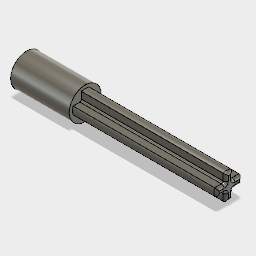
coupler2.0 v6 (Autodesk Fusion 360 design; units mm, degrees)
Autodesk Fusion 360 part; units mm, degrees
sketch "Sketch1" plane through (0, 0, 0) normal (1, 0, 0) x (0, 0, -1)
  circle A0 centre (0, 0) radius 2.3995
  dimension "d1" = 4.799
  measures "d1" diameter of A0
extrude "Extrude1" add sketch "Sketch1" along normal blind 36
sketch "Sketch2" plane through (36, 0, 0) normal (1, 0, 0) x (0, 0, -1)
  circle A0 centre (0, 0) radius 2.3995
  line L0 (0.7, 2.3995) -> (-0.7, 2.3995)
  line L1 (-0.7, -2.3995) -> (0.7, -2.3995)
  line L2 (0.7, 2.3995) -> (-0.7, -2.3995) construction
  line L3 (-0.7, 2.3995) -> (0.7, -2.3995) construction
  line L4 (-2.3995, 0.7) -> (-2.3995, -0.7)
  line L5 (2.3995, -0.7) -> (2.3995, 0.7)
  line L6 (2.3995, 0.7) -> (-2.3995, -0.7) construction
  line L7 (-2.3995, 0.7) -> (2.3995, -0.7) construction
  line L8 (-0.7, 2.3995) -> (-0.7, 1)
  line L9 (-0.7, -1) -> (-0.7, -2.3995)
  line L10 (-2.3995, -0.7) -> (-1, -0.7)
  line L11 (1, -0.7) -> (2.3995, -0.7)
  line L12 (0.7, -2.3995) -> (0.7, -1)
  line L13 (0.7, 1) -> (0.7, 2.3995)
  line L14 (2.3995, 0.7) -> (1, 0.7)
  line L15 (-1, 0.7) -> (-2.3995, 0.7)
  arc A1 (-1, 0.7) -> (-0.7, 1) centre (-1, 1) ccw
  arc A2 (0.7, 1) -> (1, 0.7) centre (1, 1) ccw
  arc A3 (1, -0.7) -> (0.7, -1) centre (1, -1) ccw
  arc A4 (-0.7, -1) -> (-1, -0.7) centre (-1, -1) ccw
  dimension "d4" = 4.799
  dimension "d5" = 1.4
  dimension "d6" = 4.799
  dimension "d7" = 1.4
  dimension "d8" = 0.3
  dimension "d11" = 0.3
  measures "d4" distance of L0.end L1.start
  measures "d5" distance of L1.start L1.end
  measures "d6" distance of L4.end L5.start
  measures "d7" distance of L4.start L4.end
  measures "d8" radius of A1
  measures "d11" radius of A4
extrude "Extrude2" cut sketch "Sketch2" against normal blind 27 contours A0 L13 L14 A2 | A0 L11 L12 A3 | A0 L8 L15 A1 | A0 L9 L10 A4
sketch "Sketch4" plane through (0, 0, 0) normal (-1, 0, 0) x (0, 0, 1)
  circle A0 centre (0, 0) radius 2.3995
  circle A1 centre (0, 0) radius 2.3995
  arc A2 (2.2951, 0.7) -> (0.7, 2.2951) centre (0, 0) ccw
extrude "Extrude4" cut sketch "Sketch4" against normal blind 9
sketch "Sketch5" plane through (9, 0, 0) normal (-1, 0, 0) x (0, 0, 1)
  line L0 (-2.2951, -0.7) -> (-1, -0.7)
  arc A0 (-0.7, -1) -> (-1, -0.7) centre (-1, -1) ccw
  line L1 (-0.7, -1) -> (-0.7, -2.2951)
  arc A1 (-0.7, -2.2951) -> (0.7, -2.2951) centre (0, 0) ccw
  line L2 (0.7, -2.2951) -> (0.7, -1)
  arc A2 (1, -0.7) -> (0.7, -1) centre (1, -1) ccw
  line L3 (1, -0.7) -> (2.2951, -0.7)
  arc A3 (2.2951, -0.7) -> (2.2951, 0.7) centre (0, 0) ccw
  line L4 (2.2951, 0.7) -> (1, 0.7)
  arc A4 (0.7, 1) -> (1, 0.7) centre (1, 1) ccw
  line L5 (0.7, 1) -> (0.7, 2.2951)
  arc A5 (0.7, 2.2951) -> (-0.7, 2.2951) centre (0, 0) ccw
  line L6 (-0.7, 2.2951) -> (-0.7, 1)
  arc A6 (-1, 0.7) -> (-0.7, 1) centre (-1, 1) ccw
  line L7 (-1, 0.7) -> (-2.2951, 0.7)
  arc A7 (-2.2951, 0.7) -> (-2.2951, -0.7) centre (0, 0) ccw
  circle A8 centre (0, 0) radius 3
  dimension "d19" = 6
  measures "d19" diameter of A8
extrude "Extrude5" add sketch "Sketch5" along normal blind 11 contours L0 A0 L1 A1 L2 A2 L3 A3 L4 A4 L5 A5 L6 A6 L7 A7 | A8
sketch "Sketch6" plane through (-2, 0, 0) normal (-1, 0, 0) x (0, 0, 1)
  circle A0 centre (0, 0) radius 3
  line L0 (-1.25, 0) -> (-1.25, 1.3297)
  line L1 (-2.2951, 0.7) -> (-1, 0.7)
  line L2 (-1.25, 1.3297) -> (-1.25, -1.3297)
  arc A1 (-1.25, -1.3297) -> (-1.25, 1.3297) centre (0, 0) ccw
  point P0 (-0.7, -2.2951)
  dimension "d22" = 3.65
  dimension "d23" = 1.25
  measures "d22" diameter of A1
  measures "d23" distance of A0.centre L0.start
extrude "Extrude6" cut sketch "Sketch6" against normal blind 9 contours L0 L2 A1
fillet "Fillet3" radius 0.5 16 edges at (36, 2.3995, 0) (36, 0.7, -1.6476) (36, 0.7879, -0.7879) (36, 1.6476, -0.7) (36, 1.6476, 0.7) (36, 0.7879, 0.7879) (36, 0.7, 1.6476) (36, 0, 2.3995) (36, -0.7, 1.6476) (36, -0.7879, 0.7879) (36, -1.6476, 0.7) (36, -2.3995, 0) (36, -1.6476, -0.7) (36, -0.7879, -0.7879) (36, -0.7, -1.6476) (36, 0, -2.3995)
